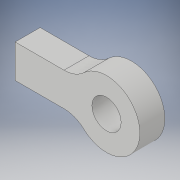
# Autodesk Inventor part: Anillo riel
Saved by Autodesk Inventor 2019 (Build 230136000, 136)
## iProperties
Created: 2020-02-01
Part Number: Anillo riel
Material: Generic
Document SubType Name: Modeling
Designer: Elías Sánchez
Density: 1 g/cm^3
Appearance: Default
Author: Elías Sánchez
Autodesk Inventor part; units mm, degrees
ref_plane "YZ Plane" through (0, 0, 0) normal (1, 0, 0) x (0, 1, 0)
ref_plane "XZ Plane" through (0, 0, 0) normal (0, 1, 0) x (-1, 0, 0)
ref_plane "XY Plane" through (0, 0, 0) normal (0, 0, 1) x (1, 0, 0)
sketch "Sketch1" plane through (0, 0, 0) normal (0, 0, 1) x (1, 0, 0)
  line L0 (0, 0) -> (15, 0)
  line L1 (15, 8) -> (0, 8)
  line L2 (0, 8) -> (0, 0)
  arc A0 (15, 0) -> (15, 8) centre (21.9282, 4) ccw
  circle A1 centre (21.9282, 4) radius 3.5
  dimension "d0" = 8
  dimension "d1" = 15
  dimension "d2" = 8
  dimension "d3" = 15
  dimension "d5" = 7
  constraints: 6 end point, 2 centre point, 2 point on circle, 1 coincident, 1 horizontal, 1 parallel, 1 vertical
  measures "d0" distance of L1.end L0.start
  measures "d1" distance of L1.start L1.end
  measures "d2" radius of A0
  measures "d3" distance of L0.start L0.end
  measures "d5" diameter of A1
extrude "Extrusion1" add sketch "Sketch1" along normal blind 6
fillet "Fillet1" radius 7 2 edges at (15, 8, 3) (15, 0, 3)
equation "\"d3\" = d1"
body "Solid1"
